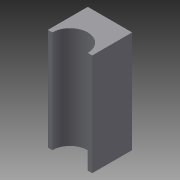
# Autodesk Inventor part: arm_block
Saved by Autodesk Inventor 2015 SP2 (Build 190223200, 223)
## iProperties
Created: 2016-09-12
Part Number: arm_block
Material: Generic
Document SubType Name: Modeling
Designer: jm799
Density: 1 g/cm^3
Appearance: Default
Author: jm799
Autodesk Inventor part; units mm, degrees
ref_plane "YZ Plane" through (0, 0, 0) normal (1, 0, 0) x (0, 1, 0)
ref_plane "XZ Plane" through (0, 0, 0) normal (0, 1, 0) x (-1, 0, 0)
ref_plane "XY Plane" through (0, 0, 0) normal (0, 0, 1) x (1, 0, 0)
sketch "Sketch1" plane through (0, 0, 0) normal (0, 1, 0) x (-1, 0, 0)
  line L0 (5, 11.4699) -> (-5, 11.4699)
  line L1 (-5, 11.4699) -> (-5, -11.5301)
  line L2 (-5, -11.5301) -> (5, -11.5301)
  line L3 (5, -11.5301) -> (5, 11.4699)
  line L4 (0, 11.4699) -> (0, -11.5301) construction
  line L5 (5, 0.0301) -> (-5, -0.0301) construction
  point P0 (0, 0)
  point P1 (0, 0)
  point P2 (0, -0.0301)
  dimension "d0" = 10
  dimension "d1" = 23
  constraints: 12 end point, 5 midpoint, 2 parallel, 1 coincident, 1 horizontal, 1 perpendicular, 1 point on line, 1 vertical alignment
  measures "d0" distance of L0.start L0.end
  measures "d1" distance of L0.end L1.end
extrude "Extrusion1" add sketch "Sketch1" along normal blind 9
sketch "Sketch4" plane through (-5, 0, 11.4699) normal (0, 0, 1) x (1, 0, 0)
  circle A0 centre (5, 0) radius 4
  dimension "d11" = 8
  constraints: 1 centre point, 1 coincident
  measures "d11" diameter of A0
hole "Hole1" at (0, 0, 11.4699) direction (0, 0, -1) diameter 8 end through all
body "Solid1"
